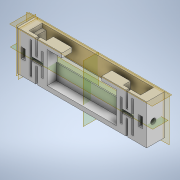
# Autodesk Inventor part: Capping_RotatingCover
Saved by Autodesk Inventor 2022 (Build 260153000, 153)
## iProperties
Created: 2024-05-06
Part Number: Capping_RotatingCover
Material: Generic
Document SubType Name: Modeling
Designer: Gotham City
Density: 1 g/cm^3
Appearance: Default
Author: Gotham City
Autodesk Inventor part; units mm, degrees
sketch "Sketch7" plane through (0, 0, 0) normal (1, 0, 0) x (0, 1, 0)
  line L0 (0, 0) -> (-20, 0)
  line L1 (-20, 0) -> (-20, 8)
  line L2 (-20, 8) -> (0, 8)
  line L3 (0, 8) -> (0, 0)
  dimension "d19" = 20
  dimension "d20" = 8
  constraints: 8 end point, 2 parallel, 1 horizontal, 1 perpendicular
  measures "d19" distance of L1.end L2.end
  measures "d20" distance of L2.end L0.start
extrude "Extrusion4" add sketch "Sketch7" along normal blind 65
sketch "Sketch8" plane through (0, -20, 8) normal (0, 0, 1) x (1, 0, 0)
  line L0 (15.15, 17.8) -> (49.85, 17.8)
  line L1 (49.85, 17.8) -> (49.85, 2.2)
  line L2 (49.85, 2.2) -> (15.15, 2.2)
  line L3 (15.15, 2.2) -> (15.15, 17.8)
  line L4 (0, 0) -> (65, 0) projected
  line L5 (0, 20) -> (65, 20) projected
  line L6 (32.5, 20) -> (32.5, 17.8) construction
  dimension "d23" = 2.2
  dimension "d24" = 34.7
  dimension "d25" = 15.6
  dimension "d77" = 2.2
  constraints: 10 end point, 2 midpoint, 2 parallel, 1 horizontal, 1 perpendicular, 1 vertical
  measures "d23" distance between parallel lines of L4 L2
  measures "d24" distance of L0.start L0.end
  measures "d25" distance of L2.end L0.start
  measures "d77" distance between parallel lines of L5 L0
extrude "Extrusion5" cut sketch "Sketch8" against normal blind 4.5
sketch "Sketch9" plane through (0, -20, 8) normal (0, 0, 1) x (1, 0, 0)
  line L0 (49.85, 2.2) -> (15.15, 2.2) construction
  line L1 (49.85, 17.8) -> (49.85, 2.2) construction
  line L2 (15.15, 17.8) -> (49.85, 17.8) construction
  line L3 (13.15, 10) -> (12.28, 10)
  line L4 (12.28, 10) -> (12.28, 4.2)
  line L5 (12.28, 4.2) -> (13.15, 4.2)
  line L6 (13.15, 4.2) -> (13.15, 10)
  line L7 (9.41, 8) -> (10.28, 8)
  line L8 (10.28, 8) -> (10.28, 0)
  line L9 (10.28, 0) -> (9.41, 0)
  line L10 (9.41, 0) -> (9.41, 8)
  line L11 (0, 0) -> (65, 0) projected
  line L12 (6.54, 10) -> (7.41, 10)
  line L13 (7.41, 10) -> (7.41, 2)
  line L14 (7.41, 2) -> (6.54, 2)
  line L15 (6.54, 2) -> (6.54, 10)
  line L16 (7.41, 10) -> (12.28, 10)
  line L17 (12.28, 10) -> (12.28, 9.13)
  line L18 (12.28, 9.13) -> (7.41, 9.13)
  line L19 (7.41, 9.13) -> (7.41, 10)
  line L20 (15.15, 2.2) -> (15.15, 17.8) projected
  line L21 (15.15, 2.2) -> (15.15, 17.8) projected
  point P0 (9.845, 8)
  point P1 (15.15, 10)
  dimension "d32" = 2
  dimension "d35" = 2
  dimension "d36" = 0.87
  dimension "d37" = 2
  dimension "d38" = 2
  dimension "d40" = 0.87
  dimension "d41" = 2
  dimension "d46" = 0.87
  dimension "d48" = 0.87
  dimension "d49" = 2
  constraints: 32 end point, 8 parallel, 4 horizontal, 4 perpendicular, 3 point on line, 2 midpoint, 1 horizontal alignment
  measures "d32" distance from line of L5 L0.end
  measures "d35" distance between parallel lines of L4 L8
  measures "d36" distance between parallel lines of L8 L10
  measures "d37" horizontal distance of L3.end L7.end
  measures "d38" distance between parallel lines of L11 L14
  measures "d40" distance between parallel lines of L13 L15
  measures "d41" distance between parallel lines of L10 L13
  measures "d46" distance between parallel lines of L16 L18
  measures "d48" distance between parallel lines of L6 L4
  measures "d49" distance between parallel lines of L20 L6
extrude "Extrusion6" cut sketch "Sketch9" against normal through all
ref_plane "Work Plane7" through (15.15, -10, 8) normal (0, -1, 0) x (1, 0, 0)
ref_plane "Work Plane6" through (32.5, 0, 0) normal (-1, 0, 0) x (0, 0, 1)
sketch "Sketch11" plane through (0, -20, 0) normal (0, 0, -1) x (-1, 0, 0)
  line L0 (0, 0) -> (-9.41, 0) projected
  line L1 (-13.15, 10) -> (-4.54, 10)
  line L2 (-4.54, 10) -> (-4.54, 0)
  line L3 (-4.54, 0) -> (-13.15, 0)
  line L4 (-13.15, 0) -> (-13.15, 10)
  line L5 (-9.41, 8) -> (-9.41, 0) projected
  line L6 (-7.41, 2) -> (-7.41, 9.13) projected
  line L7 (-6.54, 2) -> (-4.54, 2)
  line L8 (13, 10) -> (-78, 10) projected
  line L9 (-7.41, 2) -> (-6.54, 2) projected
  line L10 (-6.54, 2) -> (-7.41, 2)
  line L11 (-7.41, 9.13) -> (-7.41, 2) projected
  line L12 (-7.41, 2) -> (-7.41, 10)
  line L13 (-13.15, 10) -> (-6.54, 10) projected
  point P0 (0, 20)
  point P1 (-13.15, 4.2)
  point P2 (-7.41, 9.13)
  dimension "d42" = 2
  dimension "d47" = 2
  constraints: 14 end point, 5 point on line, 3 perpendicular, 2 horizontal, 2 parallel
  measures "d42" distance between parallel lines of L5 L6
  measures "d47" distance of L7.start L7.end
extrude "Extrusion7" cut sketch "Sketch11" against normal blind 6.5 contours L0 L3 L4 L1 L12 L6 L9 L7 L2
mirror "Mirror1" about plane through (15.15, -10, 8) normal (0, -1, 0) of "Extrusion6", "Extrusion7"
mirror "Mirror2" about plane through (32.5, 0, 0) normal (-1, 0, 0) of "Extrusion6", "Extrusion7", "Mirror1"
sketch "Sketch14" plane through (51.85, -20, 0) normal (0, 0, -1) x (-1, 0, 0)
  line L0 (38.7, 20) -> (0, 20) projected
  line L1 (0, 20) -> (0, 0) projected
  line L2 (38.7, 0) -> (0, 0) projected
  line L3 (38.7, 0) -> (38.7, 20) projected
  point P0 (51.85, 20)
extrude "Extrusion9" cut sketch "Sketch14" against normal blind 3
sketch "Sketch16" plane through (51.85, -20, 3) normal (0, 0, -1) x (-1, 0, 0)
  line L0 (0, 20) -> (38.7, 20) projected
  line L1 (29.35, 10) -> (9.35, 10)
  line L2 (9.35, 10) -> (9.35, 20)
  line L3 (9.35, 20) -> (29.35, 20)
  line L4 (29.35, 20) -> (29.35, 10)
  line L5 (19.35, 24) -> (19.35, -4) construction
  point P0 (51.85, 20)
  dimension "d55" = 20
  dimension "d56" = 10
  constraints: 8 end point, 2 parallel, 1 horizontal, 1 perpendicular, 1 point on line, 1 other
  measures "d55" distance of L1.start L1.end
  measures "d56" distance of L3.end L1.start
extrude "Extrusion10" cut sketch "Sketch16" along normal through all both and the other way through all
sketch "Sketch17" plane through (0, -20, 3.5) normal (0, 0, 1) x (1, 0, 0)
  line L0 (15.15, 17.8) -> (22.5, 17.8) projected
  line L1 (15.15, 2.2) -> (15.15, 17.8) projected
  line L2 (22.5, 17.8) -> (15.15, 17.8)
  line L3 (15.15, 17.8) -> (15.15, 10)
  line L4 (15.15, 10) -> (22.5, 10)
  line L5 (22.5, 10) -> (22.5, 17.8)
  line L6 (49.85, 17.8) -> (49.85, 2.2) projected
  line L7 (42.5, 10) -> (42.5, 20) projected
  line L8 (49.85, 17.8) -> (42.5, 17.8)
  line L9 (42.5, 17.8) -> (42.5, 10)
  line L10 (42.5, 10) -> (49.85, 10)
  line L11 (49.85, 10) -> (49.85, 17.8)
  point P0 (0, 20)
  constraints: 16 end point, 4 parallel, 2 horizontal, 2 perpendicular, 1 midpoint
extrude "Extrusion11" cut sketch "Sketch17" along normal through all both and the other way through all
sketch "Sketch18" plane through (0, 0, 0) normal (-1, 0, 0) x (0, 0, 1)
  line L0 (9.6, -10) -> (-1.6, -10) construction
  circle A0 centre (4.7, -10) radius 3.3 construction
  line L1 (8, 0) -> (8, -20) construction
  point P0 (0, 0)
  dimension "d61" = 6.6
  constraints: 1 centre point, 1 point on line, 1 tangent
  measures "d61" diameter of A0
hole "Hole1" at (0, -10, 4.7) direction (1, 0, 0) diameter 2.6 depth 6 tip angle 118 clearance for "Socket Head Cap Screw ISO 4762" size "M2.5" standard "ISO"
ref_plane "Work Plane8" through (2, 0, 0) normal (1, 0, 0) x (0, 1, 0)
sketch "Sketch19" plane through (2, 0, 0) normal (1, 0, 0) x (0, 1, 0)
  circle A0 centre (-10, 4.7) radius 1.3 construction
  circle A1 centre (-10, 4.7) radius 0.4013 projected
  line L0 (-12.55, 3.2278) -> (-12.55, 6.1722)
  line L1 (-12.55, 6.1722) -> (-10, 7.6445) construction
  line L2 (-10, 7.6445) -> (-7.45, 6.1722) construction
  line L3 (-7.45, 6.1722) -> (-7.45, 3.2278)
  line L4 (-7.45, 3.2278) -> (-10, 1.7555)
  line L5 (-10, 1.7555) -> (-12.55, 3.2278)
  line L6 (-7.45, 6.1722) -> (-7.45, 8)
  line L7 (-12.55, 6.1722) -> (-12.55, 8)
  line L8 (-12.55, 8) -> (-7.45, 8)
  line L9 (0, 8) -> (-20, 8) projected
  point P0 (0, 0)
  dimension "d70" = 5.1
  constraints: 18 end point, 2 point on line, 2 vertical, 1 coincident, 1 perpendicular, 13 other
  measures "d70" distance between parallel lines of L0 L3
extrude "Extrusion12" cut sketch "Sketch19" along normal blind 2.05
mirror "Mirror3" about plane through (32.5, 0, 0) normal (-1, 0, 0) of "Hole1", "Extrusion12"
sketch "Sketch20" plane through (0, -20, 0) normal (0, 0, -1) x (-1, 0, 0)
  line L0 (-4.54, 20) -> (-4.54, 18) projected
  line L1 (-4.54, 18) -> (-6.54, 18) projected
  line L2 (-6.54, 18) -> (-6.54, 2) projected
  line L3 (-6.54, 2) -> (-4.54, 2) projected
  line L4 (-4.54, 2) -> (-4.54, 0) projected
  line L5 (0, 0) -> (-4.54, 0) projected
  line L6 (0, 0) -> (0, 20) projected
  line L7 (0, 20) -> (-4.54, 20) projected
  line L8 (-60.46, 18) -> (-60.46, 20) projected
  line L9 (-60.46, 20) -> (-65, 20) projected
  line L10 (-65, 0) -> (-65, 20) projected
  line L11 (-60.46, 0) -> (-65, 0) projected
  line L12 (-60.46, 0) -> (-60.46, 2) projected
  line L13 (-60.46, 2) -> (-58.46, 2) projected
  line L14 (-58.46, 2) -> (-58.46, 18) projected
  line L15 (-58.46, 18) -> (-60.46, 18) projected
  line L16 (0, 20) -> (-4.54, 20) projected
  line L17 (-65, 20) -> (-65, 0) projected
  line L18 (0, 20) -> (-65, 20)
  line L19 (-65, 20) -> (-65, 10)
  line L20 (-65, 10) -> (0, 10)
  line L21 (0, 10) -> (0, 20)
  line L22 (-65, 0) -> (-65, 20) projected
  line L23 (-65, 11) -> (0, 11)
  point P0 (-6.54, 10)
  point P1 (-58.46, 10)
  point P2 (-58.46, 11)
  point P3 (-6.54, 11)
  dimension "d78" = 1
  constraints: 10 end point, 2 parallel, 2 perpendicular, 2 point on line, 1 horizontal, 1 midpoint
  measures "d78" distance between parallel lines of L20 L23
extrude "Extrusion13" add sketch "Sketch20" along normal blind 1 contours L7 L6 L23 L2 L1 L0 | L0 L1 L2 L23 L14 L15 L8 L18 | L8 L15 L14 L23 L10 L9 | L6 L20 L2 L23 | L6 L5 L4 L3 L2 L20 | L23 L14 L20 L10 | L20 L14 L13 L12 L11 L10
thicken "Thicken2" operation add thickness 0.035 both sides no extend neighbours yes toward (0, -1, 0) faces at (26.7167, -17.8, 6.5) (15.15, -10, 6.5) (20.05, -2.2, 6.3333) (49.85, -10, 6.5) (47.4, -2.2, 6.3333)
equation "\"d77\" = d23"
equation "\"d36\" = d48"
equation "\"d37\" = d32"
equation "\"d38\" = d37"
equation "\"d40\" = d48"
equation "\"d41\" = d35"
equation "\"d46\" = d48"
equation "\"d47\" = d42"
body "Solid1"
body "Solid2"
